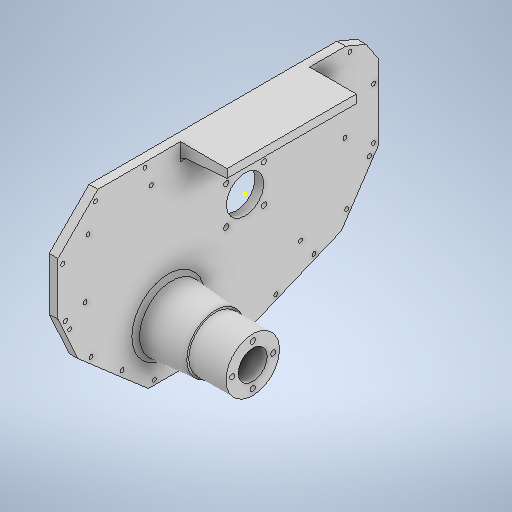
# Autodesk Inventor part: body_side_R2
Saved by Autodesk Inventor 2025.2 (Build 292293000, 293)
## iProperties
Created: 2025-04-13
Part Number: body_side_R2
Material: Generic
Document SubType Name: Modeling
Designer: Bruno
Density: 1 g/cm^3
Appearance: Default
Author: Bruno
## iProperties of the stored document body_side_R2_3DPrint.ipt
Created: 2025-05-06
Part Number: body_side_R2_3DPrint
Material: Generic
Document SubType Name: Modeling
Designer: Bruno
Density: 1 g/cm^3
Appearance: Default
Author: Bruno
Autodesk Inventor part; units mm, degrees
ref_plane "YZ Plane" through (0, 0, 0) normal (1, 0, 0) x (0, 1, 0)
ref_plane "XZ Plane" through (0, 0, 0) normal (0, 1, 0) x (-1, 0, 0)
ref_plane "XY Plane" through (0, 0, 0) normal (0, 0, 1) x (1, 0, 0)
sketch "Sketch1" plane through (0, 0, 0) normal (1, 0, 0) x (0, 1, 0)
  line L0 (0, 0) -> (-50.1885, 57.7353) construction
  line L1 (0, 0) -> (0, 3.0029) construction
  circle A0 centre (0, 0) radius 20 construction
  circle A1 centre (-14.1421, 14.1421) radius 2
  line L2 (-14.1421, 14.1421) -> (0, 0) construction
  circle A2 centre (-14.1421, -14.1421) radius 2
  circle A3 centre (14.1421, -14.1421) radius 2
  circle A4 centre (14.1421, 14.1421) radius 2
  circle A5 centre (-50.1885, 57.7353) radius 19 construction
  line L3 (-90, 0) -> (-90, 72.6202)
  line L4 (-90, 72.6202) -> (-31.0219, 140.4668)
  line L5 (-31.0219, 140.4668) -> (90, 140.4668)
  line L6 (90, 140.4668) -> (90, 0)
  line L7 (-80.2346, 83.854) -> (-64.528, 70.2004) construction
  line L8 (-90, 57.7353) -> (-69.1885, 57.7353) construction
  circle A6 centre (-34.7385, 57.7353) radius 3.55
  circle A7 centre (-50.1885, 73.1853) radius 3.55
  circle A8 centre (-65.6385, 57.7353) radius 3.55
  circle A9 centre (-50.1885, 42.2853) radius 3.55
  line L9 (-46.6385, 73.1853) -> (-46.6385, 67.9881)
  line L10 (-53.7385, 73.1853) -> (-53.7385, 67.9881)
  line L11 (-65.6385, 61.2853) -> (-60.4413, 61.2853)
  line L12 (-65.6385, 54.1853) -> (-60.4413, 54.1853)
  line L13 (-53.7385, 42.2853) -> (-53.7385, 47.4825)
  line L14 (-46.6385, 42.2853) -> (-46.6385, 47.4825)
  line L15 (-34.7385, 54.1853) -> (-39.9357, 54.1853)
  line L16 (-34.7385, 61.2853) -> (-39.9357, 61.2853)
  arc A10 (-39.9357, 61.2853) -> (-46.6385, 67.9881) centre (-50.1885, 57.7353) ccw
  arc A11 (-46.6385, 47.4825) -> (-39.9357, 54.1853) centre (-50.1885, 57.7353) ccw
  arc A12 (-53.7385, 67.9881) -> (-60.4413, 61.2853) centre (-50.1885, 57.7353) ccw
  arc A13 (-60.4413, 54.1853) -> (-53.7385, 47.4825) centre (-50.1885, 57.7353) ccw
  circle A14 centre (0, 0) radius 14
  line L17 (90, 0) -> (61.1538, -69.2308)
  line L18 (-90, 0) -> (-61.1538, -69.2308)
  circle A15 centre (0, 0) radius 46 construction
  line L19 (15, -100) -> (-15, -100)
  arc A16 (15, -100) -> (61.1538, -69.2308) centre (15, -50) ccw
  arc A17 (-61.1538, -69.2308) -> (-15, -100) centre (-15, -50) ccw
  line L20 (-50.1885, 57.7353) -> (32.543, 140.4668) construction
  line L21 (61.1538, -69.2308) -> (48.3333, -100)
  line L22 (15, -100) -> (48.3333, -100)
  line L23 (-15, -100) -> (-48.3333, -100)
  line L24 (-48.3333, -100) -> (-61.1538, -69.2308)
  point P0 (-34.7385, 61.2853)
  point P1 (-34.7385, 54.1853)
  point P2 (-46.6385, 42.2853)
  point P3 (-53.7385, 42.2853)
  point P4 (-65.6385, 54.1853)
  point P5 (-65.6385, 61.2853)
  dimension "d2" = 40
  dimension "d0" = 41
  dimension "d1" = 76.5
  dimension "d3" = 4
  dimension "d8" = 45
  dimension "d11" = 360
  dimension "d14" = 41
  dimension "d18" = 7.1
  dimension "d21" = 360
  dimension "d26" = 360
  dimension "d28" = 10.85
  dimension "d29" = 28
  dimension "d52" = 30.9
  dimension "d66" = 180
  dimension "d67" = 90
  dimension "d68" = 92
  dimension "d85" = 100
  dimension "d86" = 50
  dimension "d87" = 30
  dimension "d88" = 117
  dimension "d89" = 45
  constraints: 50 end point, 17 centre point, 17 point on circle, 10 tangent, 5 horizontal, 5 vertical, 4 coincident, 3 horizontal alignment, 3 point on line, 2 equal length, 2 line through centre, 1 equal radius, 1 perpendicular, 47 other
  measures "d0" angle of L1 L0
  measures "d1" distance of L0.end L0.start
  measures "d3" diameter of A1
  measures "d8" angle of L1 L2
  measures "d14" angle of L4 L3
  measures "d18" diameter of A6
  measures "d28" radius of A10
  measures "d29" diameter of A14
  measures "d52" distance of A9.centre A7.centre
  measures "d66" distance of L6.end L3.start
  measures "d67" distance from line of L6 A14.centre
  measures "d68" diameter of A15
  measures "d85" distance from line of L6.end L19
  measures "d86" radius of A16
  measures "d87" distance of A16.centre A17.centre
  measures "d88" distance of L20.start L20.end
  measures "d89" angle of L3 L20
extrude "Extrusion1" add sketch "Sketch1" along normal blind 6.6
sketch "Sketch2" plane through (0, 0, 0) normal (-1, 0, 0) x (0, 0, 1)
  arc A0 (54.1853, -39.9357) -> (47.4825, -46.6385) centre (57.7353, -50.1885) ccw projected
  circle A1 centre (57.7353, -50.1885) radius 21.5
  point P0 (0, 0)
  point P1 (52.1533, -40.4479)
  point P2 (48.8897, -44.3373)
  dimension "d35" = 43
  constraints: 1 centre point, 1 coincident
  measures "d35" diameter of A1
extrude "Extrusion2" add sketch "Sketch2" along normal blind 35.5
chamfer "Chamfer1" distance 3 distance2 35.5 1 edges at (0, -50.1885, 36.2353) measured on face at (0, -50.1885, 35.7353)
fillet "Fillet1" radius 3 1 edges at (0, -50.1885, 33.2354)
sketch "Sketch3" plane through (-35.5, -50.1885, 57.7353) normal (-1, 0, 0) x (0, 0, 1)
  circle A0 centre (0, 0) radius 21.5 projected
  circle A1 centre (0, 0) radius 20.05
  point P0 (-57.7353, 50.1885)
  dimension "d40" = 40.1
  constraints: 1 centre point, 1 coincident
  measures "d40" diameter of A1
extrude "Extrusion3" add sketch "Sketch3" along normal blind 28 contours A1
sketch "Sketch4" plane through (0, 0, 0) normal (1, 0, 0) x (0, 0, -1)
  arc A0 (-47.4825, -46.6385) -> (-54.1853, -39.9357) centre (-57.7353, -50.1885) ccw projected
  circle A1 centre (-57.7353, -50.1885) radius 10.85
  arc A2 (-47.4825, -46.6385) -> (-54.1853, -39.9357) centre (-57.7353, -50.1885) ccw projected
  point P0 (0, 0)
  point P1 (-54.1853, -39.9357)
  point P2 (-47.4825, -46.6385)
  point P3 (-48.8897, -44.3373)
  point P4 (-52.1533, -40.4479)
  constraints: 1 centre point, 1 coincident, 1 concentric
extrude "Extrusion4" cut sketch "Sketch4" against normal through all
sketch "Sketch5" plane through (0, 0, 0) normal (1, 0, 0) x (0, 0, -1)
  arc A0 (-42.2853, -53.7385) -> (-42.2853, -46.6385) centre (-42.2853, -50.1885) ccw projected
  circle A1 centre (-42.2853, -50.1885) radius 2
  arc A2 (-54.1853, -60.4413) -> (-47.4825, -53.7385) centre (-57.7353, -50.1885) ccw projected
  circle A3 centre (-57.7353, -34.7385) radius 2
  circle A4 centre (-73.1853, -50.1885) radius 2
  circle A5 centre (-57.7353, -65.6385) radius 2
  point P0 (0, 0)
  dimension "d45" = 4
  dimension "d48" = 360
  constraints: 4 centre point, 1 coincident, 9 other
  measures "d45" diameter of A1
extrude "Extrusion5" cut sketch "Sketch5" against normal through all
sketch "Sketch6" plane through (0, 0, 0) normal (1, 0, 0) x (0, 0, -1)
  circle A0 centre (-57.7353, -65.6385) radius 2 projected
  circle A1 centre (-57.7353, -65.6385) radius 2 projected
  arc A2 (-61.2853, -60.4413) -> (-54.1853, -60.4413) centre (-57.7353, -50.1885) ccw projected
  line L0 (-61.2853, -65.6385) -> (-61.2853, -60.4413) projected
  arc A3 (-61.2853, -65.6385) -> (-54.1853, -65.6385) centre (-57.7353, -65.6385) ccw projected
  line L1 (-54.1853, -60.4413) -> (-54.1853, -65.6385) projected
  circle A4 centre (-42.2853, -50.1885) radius 2 projected
  arc A5 (-47.4825, -53.7385) -> (-47.4825, -46.6385) centre (-57.7353, -50.1885) ccw projected
  line L2 (-42.2853, -53.7385) -> (-47.4825, -53.7385) projected
  arc A6 (-42.2853, -53.7385) -> (-42.2853, -46.6385) centre (-42.2853, -50.1885) ccw projected
  line L3 (-47.4825, -46.6385) -> (-42.2853, -46.6385) projected
  circle A7 centre (-57.7353, -34.7385) radius 2 projected
  arc A8 (-54.1853, -39.9357) -> (-61.2853, -39.9357) centre (-57.7353, -50.1885) ccw projected
  line L4 (-54.1853, -34.7385) -> (-54.1853, -39.9357) projected
  arc A9 (-54.1853, -34.7385) -> (-61.2853, -34.7385) centre (-57.7353, -34.7385) ccw projected
  line L5 (-61.2853, -39.9357) -> (-61.2853, -34.7385) projected
  circle A10 centre (-73.1853, -50.1885) radius 2 projected
  arc A11 (-67.9881, -46.6385) -> (-67.9881, -53.7385) centre (-57.7353, -50.1885) ccw projected
  line L6 (-73.1853, -46.6385) -> (-67.9881, -46.6385) projected
  arc A12 (-73.1853, -46.6385) -> (-73.1853, -53.7385) centre (-73.1853, -50.1885) ccw projected
  line L7 (-67.9881, -53.7385) -> (-73.1853, -53.7385) projected
  line L8 (-42.2853, -53.7385) -> (-47.4825, -53.7385) projected
  arc A13 (-42.2853, -53.7385) -> (-42.2853, -46.6385) centre (-42.2853, -50.1885) ccw projected
  line L9 (-47.4825, -46.6385) -> (-42.2853, -46.6385) projected
  arc A14 (-47.4825, -53.7385) -> (-47.4825, -46.6385) centre (-57.7353, -50.1885) ccw projected
  arc A15 (-61.2853, -60.4413) -> (-54.1853, -60.4413) centre (-57.7353, -50.1885) ccw projected
  line L10 (-61.2853, -65.6385) -> (-61.2853, -60.4413) projected
  arc A16 (-61.2853, -65.6385) -> (-54.1853, -65.6385) centre (-57.7353, -65.6385) ccw projected
  line L11 (-54.1853, -60.4413) -> (-54.1853, -65.6385) projected
  arc A17 (-67.9881, -46.6385) -> (-67.9881, -53.7385) centre (-57.7353, -50.1885) ccw projected
  line L12 (-73.1853, -46.6385) -> (-67.9881, -46.6385) projected
  arc A18 (-73.1853, -46.6385) -> (-73.1853, -53.7385) centre (-73.1853, -50.1885) ccw projected
  line L13 (-67.9881, -53.7385) -> (-73.1853, -53.7385) projected
  arc A19 (-54.1853, -39.9357) -> (-61.2853, -39.9357) centre (-57.7353, -50.1885) ccw projected
  line L14 (-54.1853, -34.7385) -> (-54.1853, -39.9357) projected
  arc A20 (-54.1853, -34.7385) -> (-61.2853, -34.7385) centre (-57.7353, -34.7385) ccw projected
  line L15 (-61.2853, -39.9357) -> (-61.2853, -34.7385) projected
  arc A21 (-61.2853, -60.4413) -> (-54.1853, -60.4413) centre (-57.7353, -50.1885) ccw projected
  line L16 (-61.2853, -65.6385) -> (-61.2853, -60.4413) projected
  arc A22 (-61.2853, -65.6385) -> (-54.1853, -65.6385) centre (-57.7353, -65.6385) ccw projected
  line L17 (-54.1853, -60.4413) -> (-54.1853, -65.6385) projected
  arc A23 (-67.9881, -46.6385) -> (-67.9881, -53.7385) centre (-57.7353, -50.1885) ccw projected
  line L18 (-73.1853, -46.6385) -> (-67.9881, -46.6385) projected
  arc A24 (-73.1853, -46.6385) -> (-73.1853, -53.7385) centre (-73.1853, -50.1885) ccw projected
  line L19 (-67.9881, -53.7385) -> (-73.1853, -53.7385) projected
  point P0 (0, 0)
extrude "Extrusion6" cut sketch "Sketch6" against normal blind 20.5 contours A0 | A2 L1 A3 L0 | A4 | A5 L3 A6 L2 | A8 L5 A9 L4 | A11 L7 A12 L6
sketch "Sketch7" plane through (6.6, 0, 0) normal (1, 0, 0) x (0, 0, -1)
  circle A0 centre (0, 0) radius 14 projected
  line L0 (0, 14) -> (0, 32) construction
  line L1 (0, 32) -> (3, 32) construction
  line L2 (0, 38) -> (3, 38) construction
  arc A1 (3, 32) -> (3, 38) centre (3, 35) ccw construction
  line L3 (0, 32) -> (-3, 32) construction
  line L4 (0, 38) -> (-3, 38) construction
  arc A2 (-3, 38) -> (-3, 32) centre (-3, 35) ccw construction
  line L5 (-3, 39.5) -> (0, 39.5)
  line L6 (0, 39.5) -> (3, 39.5)
  arc A3 (3, 30.5) -> (3, 39.5) centre (3, 35) ccw
  line L7 (3, 30.5) -> (0, 30.5)
  line L8 (0, 30.5) -> (-3, 30.5)
  arc A4 (-3, 39.5) -> (-3, 30.5) centre (-3, 35) ccw
  dimension "d55" = 18
  dimension "d56" = 3
  dimension "d57" = 6
  dimension "d58" = 1.5
  constraints: 18 end point, 8 point on circle, 4 centre point, 3 symmetric about line, 2 horizontal, 2 tangent, 2 vertical alignment, 1 vertical, 7 other
  measures "d55" distance of L0.start L0.end
  measures "d56" distance of L0.end L1.end
  measures "d57" distance between parallel lines of L2 L1
  measures "d58" distance between parallel lines of L4 L5
extrude "Extrusion7" cut sketch "Sketch7" against normal through all contours L5 L6 A3 L7 L8 A4
sketch "Sketch8" plane through (6.6, 0, 0) normal (1, 0, 0) x (0, 0, -1)
  circle A0 centre (-30, 22) radius 2.225
  circle A1 centre (0, 0) radius 14 projected
  line L0 (0, 0) -> (-5.1199, 0) construction
  line L1 (0, 0) -> (0, 4.2837) construction
  circle A2 centre (-30, -22) radius 2.225
  circle A3 centre (30, 22) radius 2.225
  circle A4 centre (30, -22) radius 2.225
  dimension "d61" = 4.45
  dimension "d62" = 30
  dimension "d63" = 22
  constraints: 4 centre point, 4 end point, 3 symmetric about line, 1 horizontal, 1 vertical, 3 other
  measures "d61" diameter of A0
  measures "d62" horizontal distance of A0.centre L0.start
  measures "d63" vertical distance of A0.centre L0.start
extrude "Extrusion8" cut sketch "Sketch8" against normal blind 6 contours A0 | A2 | A3 | A4
sketch "Sketch13" plane through (6.6, 0, 0) normal (1, 0, 0) x (0, 0, -1)
  circle A0 centre (0, 0) radius 14 projected
  circle A1 centre (0, 0) radius 46 construction
  line L0 (0, 103.5) -> (0, 58.5) construction
  line L1 (-26, 58.5) -> (26, 58.5)
  line L2 (25.1057, 48.5) -> (-25.1057, 48.5) construction
  line L3 (0, 46) -> (0, 48.5) construction
  line L4 (0, 90) -> (-140.4668, 90) projected
  line L5 (-26, 58.5) -> (-26, 90)
  line L6 (26, 58.5) -> (26, 79.1667)
  line L7 (-140.4668, 90) -> (-140.4668, -31.0219) projected
  line L8 (26, 58.5) -> (75.6, 58.5)
  line L9 (-26, 58.5) -> (-140.4668, 58.5)
  line L10 (100, 48.3333) -> (0, 90) projected
  dimension "d90" = 92
  dimension "d91" = 45
  dimension "d92" = 52
  dimension "d93" = 10
  dimension "d94" = 2.5
  constraints: 16 end point, 4 vertical alignment, 3 horizontal, 3 point on line, 3 vertical, 2 midpoint, 2 perpendicular, 1 coincident, 2 other
  measures "d91" distance of L0.start L0.end
  measures "d92" distance of L1.start L1.end
  measures "d93" distance between parallel lines of L1 L2
  measures "d94" distance of L3.start L3.end
extrude "Extrusion9" cut sketch "Sketch13" against normal blind 10 contours L5 L4 L10 L6 L1 | L9 L7 L4 L5 | L6 L10 L8
sketch "Sketch15" plane through (0, 0, 0) normal (-1, 0, 0) x (0, 0, 1)
  point P0 (0, 0)
chamfer "Chamfer2" distance 30 angle 45 2 edges at (3.3, -48.3333, -100) (3.3, 58.5, 140.4668)
chamfer "Chamfer3" distance 20 angle 45 1 edges at (3.3, -31.0219, 140.4668)
chamfer "Chamfer4" distance 10 angle 45 1 edges at (3.3, 48.3333, -100)
sketch "Sketch16" plane through (0, 0, 0) normal (-1, 0, 0) x (0, 0, 1)
  line L0 (-100, 38.3333) -> (-90.7692, 52.1795) projected
  line L1 (-100, -18.3333) -> (-100, 38.3333) projected
  line L2 (-72.3077, -59.8718) -> (-100, -18.3333) projected
  line L3 (0, -90) -> (-72.3077, -59.8718) projected
  line L4 (72.6202, -90) -> (0, -90) projected
  line L5 (125.3726, -44.143) -> (72.6202, -90) projected
  line L6 (140.4668, -11.0219) -> (125.3726, -44.143) projected
  line L7 (140.4668, 28.5) -> (140.4668, -11.0219) projected
  line L8 (110.4668, 58.5) -> (140.4668, 28.5) projected
  line L9 (110.4668, 58.5) -> (-75.6, 58.5) projected
  line L10 (-90.7692, 52.1795) -> (-75.6, 58.5) projected
  arc A0 (3, 30.5) -> (3, 39.5) centre (3, 35) ccw projected
  line L11 (3, 30.5) -> (-3, 30.5) projected
  arc A1 (-3, 39.5) -> (-3, 30.5) centre (-3, 35) ccw projected
  line L12 (-3, 39.5) -> (3, 39.5) projected
  circle A2 centre (14.1421, -14.1421) radius 2 projected
  circle A3 centre (-14.1421, -14.1421) radius 2 projected
  circle A4 centre (-14.1421, 14.1421) radius 2 projected
  circle A5 centre (14.1421, 14.1421) radius 2 projected
  circle A6 centre (0, 0) radius 14 projected
  circle A7 centre (57.7353, -50.1885) radius 27.2572 projected
  line L13 (-90.7692, 52.1795) -> (116.7873, 52.1795)
  circle A8 centre (0, 0) radius 46 construction
  circle A9 centre (0, 0) radius 48.5
  line L14 (-48.5, 0) -> (-48.5, 58.5)
  line L15 (48.5, 0) -> (48.5, 58.5)
  point P0 (48.5, 52.1795)
  point P1 (-48.5, 52.1795)
  dimension "d115" = 92
  dimension "d116" = 2.5
  constraints: 6 end point, 3 point on line, 2 centre point, 2 coincident, 2 perpendicular, 2 point on circle, 2 tangent, 1 horizontal
  measures "d115" diameter of A8
  measures "d116" radial gap between concentric circles of A8 A9
extrude "Extrusion11" add sketch "Sketch16" along normal blind 35 contours L14 L9 L15 L13
sketch "Sketch18" plane through (6.6, 0, 0) normal (1, 0, 0) x (0, 0, -1)
  circle A0 centre (96.475, 23.7415) radius 1.5 projected
  circle A1 centre (96.475, 23.7415) radius 1.5 projected
  circle A2 centre (96.475, -14.8083) radius 1.5 projected
  circle A3 centre (93.4135, -21.8583) radius 1.5 projected
  circle A4 centre (76.1956, -47.6852) radius 1.5 projected
  circle A5 centre (51.6799, -64.648) radius 1.5 projected
  circle A6 centre (23.0276, -76.5864) radius 1.5 projected
  circle A7 centre (-6.0346, -86.475) radius 1.5 projected
  circle A8 centre (-37.0746, -86.475) radius 1.5 projected
  circle A9 centre (-68.1146, -86.475) radius 1.5 projected
  circle A10 centre (-92.3227, -68.2022) radius 1.5 projected
  circle A11 centre (-115.7488, -47.8382) radius 1.5 projected
  circle A12 centre (-131.6545, -21.8583) radius 1.5 projected
  circle A13 centre (-134.8674, -14.8083) radius 1.5 projected
  circle A14 centre (-136.9418, 23.2911) radius 1.5 projected
  circle A15 centre (-112.3337, 51.6479) radius 1.5 projected
  circle A16 centre (-75.162, 54.975) radius 1.5 projected
  circle A17 centre (-36.6122, 54.975) radius 1.5 projected
  circle A18 centre (1.9376, 54.975) radius 1.5 projected
  circle A19 centre (40.4874, 54.975) radius 1.5 projected
  circle A20 centre (78.7186, 53.3818) radius 1.5 projected
  circle A21 centre (-134.8674, -14.8083) radius 1.65
  point P0 (0, 0)
  dimension "d117" = 3.3
  constraints: 1 centre point, 1 coincident
  measures "d117" diameter of A21
extrude "Extrusion12" cut sketch "Sketch18" against normal through all contours A0 | A2 | A3 | A4 | A5 | A6 | A7 | A8 | A9 | A10 | A11 | A12 | A13 | A14 | A15 | A16 | A20 | A21
chamfer "Chamfer5" distance 3 distance2 35 1 edges at (0, 52.1795, 0) measured on face at (0, 51.6795, 0)
fillet "Fillet5" radius 4 1 edges at (0, 49.1796, 0)
sketch "Sketch19" plane through (6.6, 0, 0) normal (1, 0, 0) x (0, 0, -1)
  circle A0 centre (60.0011, 43.3256) radius 2.225 projected
  circle A1 centre (41.5764, -50.8737) radius 2.225 projected
  circle A2 centre (74.9972, -0.7443) radius 2.225 projected
  circle A3 centre (96.475, 23.7415) radius 2.8 projected
  circle A4 centre (51.6799, -64.648) radius 2.8 projected
  circle A5 centre (96.475, -14.8083) radius 2.8 projected
  circle A6 centre (78.7186, 53.3818) radius 2.8 projected
  circle A7 centre (76.1956, -47.6852) radius 2.8 projected
  circle A8 centre (93.4135, -21.8583) radius 2.8 projected
  arc A9 (30.8564, -39.3432) -> (27.0276, -47.2118) centre (37.0276, -47.2118) ccw projected
  line L0 (27.0276, -78.7385) -> (27.0276, -47.2118) projected
  line L1 (72.3077, -59.8718) -> (27.0276, -78.7385) projected
  line L2 (100, -18.3333) -> (72.3077, -59.8718) projected
  line L3 (100, 38.3333) -> (100, -18.3333) projected
  line L4 (90.7692, 52.1795) -> (100, 38.3333) projected
  line L5 (75.6, 58.5) -> (90.7692, 52.1795) projected
  line L6 (48.5, 58.5) -> (75.6, 58.5) projected
  line L7 (48.5, 45.5077) -> (48.5, 58.5) projected
  line L8 (32.8444, 41.8922) -> (48.5, 45.5077) projected
  arc A10 (32.8444, 41.8922) -> (32.0139, 38.4072) centre (33.2944, 39.9435) ccw projected
  arc A11 (30.8564, -39.3432) -> (32.0139, 38.4072) centre (0, 0) ccw projected
  circle A12 centre (-120.1367, -10.0647) radius 2.225 projected
  circle A13 centre (-117.9117, 32.9479) radius 2.225 projected
  circle A14 centre (-70.353, 41.1006) radius 2.225 projected
  circle A15 centre (-136.9418, 23.2911) radius 2.8 projected
  circle A16 centre (-112.3337, 51.6479) radius 2.8 projected
  circle A17 centre (-134.8674, -14.8083) radius 2.8 projected
  circle A18 centre (-75.162, 54.975) radius 2.8 projected
  circle A19 centre (-131.6545, -21.8583) radius 2.8 projected
  arc A20 (-42.1883, 31.8997) -> (-35.8142, 34.8905) centre (-42.977, 41.8686) ccw projected
  arc A21 (-32.0139, 38.4072) -> (-35.8142, 34.8905) centre (0, 0) ccw projected
  arc A22 (-32.0139, 38.4072) -> (-32.8444, 41.8922) centre (-33.2944, 39.9435) ccw projected
  line L9 (-48.5, 45.5077) -> (-32.8444, 41.8922) projected
  line L10 (-48.5, 58.5) -> (-48.5, 45.5077) projected
  line L11 (-110.4668, 58.5) -> (-48.5, 58.5) projected
  line L12 (-140.4668, 28.5) -> (-110.4668, 58.5) projected
  line L13 (-140.4668, -11.0219) -> (-140.4668, 28.5) projected
  line L14 (-125.3726, -44.143) -> (-140.4668, -11.0219) projected
  line L15 (-87.7648, 23.7979) -> (-125.3726, -44.143) projected
  arc A23 (-79.8044, 28.9239) -> (-87.7648, 23.7979) centre (-79.0157, 18.955) ccw projected
  line L16 (-42.1883, 31.8997) -> (-79.8044, 28.9239) projected
  circle A24 centre (-70.353, 41.1006) radius 1.5
  circle A25 centre (-117.9117, 32.9479) radius 1.5
  circle A26 centre (-120.1367, -10.0647) radius 1.5
  circle A27 centre (60.0011, 43.3256) radius 1.5
  circle A28 centre (74.9972, -0.7443) radius 1.5
  circle A29 centre (41.5764, -50.8737) radius 1.5
  point P0 (0, 0)
  dimension "d124" = 3
  dimension "d125" = 3
  dimension "d126" = 3
  dimension "d127" = 3
  dimension "d128" = 3
  dimension "d129" = 3
  constraints: 6 centre point, 6 coincident
  measures "d124" diameter of A24
  measures "d125" diameter of A25
  measures "d126" diameter of A26
  measures "d127" diameter of A27
  measures "d128" diameter of A28
  measures "d129" diameter of A29
extrude "Extrusion13" cut sketch "Sketch19" against normal through all contours A24 | A25 | A26 | A27 | A28 | A29
sketch "Sketch20" plane through (6.6, 0, 0) normal (1, 0, 0) x (0, 0, -1)
  circle A0 centre (-117.9117, 32.9479) radius 1.5 projected
  circle A1 centre (-117.9117, 32.9479) radius 2.8
  circle A2 centre (-70.353, 41.1006) radius 1.5 projected
  circle A3 centre (-70.353, 41.1006) radius 2.8
  circle A4 centre (-120.1367, -10.0647) radius 1.5 projected
  circle A5 centre (-120.1367, -10.0647) radius 2.8
  circle A6 centre (60.0011, 43.3256) radius 1.5 projected
  circle A7 centre (60.0011, 43.3256) radius 2.8
  circle A8 centre (74.9972, -0.7443) radius 1.5 projected
  circle A9 centre (74.9972, -0.7443) radius 2.8
  circle A10 centre (41.5764, -50.8737) radius 1.5 projected
  circle A11 centre (41.5764, -50.8737) radius 2.8
  point P0 (0, 0)
  dimension "d132" = 5.6
  dimension "d133" = 5.6
  dimension "d134" = 5.6
  dimension "d135" = 5.6
  dimension "d136" = 5.6
  dimension "d137" = 5.6
  constraints: 6 centre point, 6 coincident
  measures "d132" diameter of A1
  measures "d133" diameter of A3
  measures "d134" diameter of A5
  measures "d135" diameter of A7
  measures "d136" diameter of A9
  measures "d137" diameter of A11
extrude "Extrusion14" cut sketch "Sketch20" against normal blind 3 contours A1 | A3 | A4 | A5 | A6 | A7 | A8 | A9 | A11
mirror "Mirror1" about plane through (0, 0, 0) normal (1, 0, 0) remove original yes
sketch "Sketch21" plane through (-6.6, -18.3333, -100) normal (-1, 0, 0) x (0, 0, 1)
  circle A0 centre (85.8579, 32.4755) radius 2 projected
  circle A1 centre (85.8579, 32.4755) radius 3.55
  circle A2 centre (114.1421, 32.4755) radius 2 projected
  circle A3 centre (114.1421, 32.4755) radius 3.55
  circle A4 centre (114.1421, 4.1912) radius 2 projected
  circle A5 centre (114.1421, 4.1912) radius 3.55
  circle A6 centre (85.8579, 4.1912) radius 2 projected
  circle A7 centre (85.8579, 4.1912) radius 3.55
  point P0 (100, 18.3333)
  dimension "d140" = 7.1
  dimension "d141" = 7.1
  dimension "d142" = 7.1
  dimension "d143" = 7.1
  constraints: 4 centre point, 4 coincident
  measures "d140" diameter of A1
  measures "d141" diameter of A3
  measures "d142" diameter of A5
  measures "d143" diameter of A7
extrude "Extrusion15" cut sketch "Sketch21" against normal blind 2 contours A0 | A1 | A2 | A3 | A4 | A5 | A6 | A7
sketch "Sketch22" plane through (20.5, -39.9357, 61.2853) normal (-1, 0, 0) x (0, 0, 1)
  circle A0 centre (-3.55, 5.1972) radius 2 projected
  line L0 (0, 0) -> (0, 5.1972) projected
  arc A1 (0, 5.1972) -> (-7.1, 5.1972) centre (-3.55, 5.1972) ccw projected
  line L1 (-7.1, 5.1972) -> (-7.1, 0) projected
  arc A2 (0, 0) -> (-7.1, 0) centre (-3.55, -10.2528) ccw projected
  circle A3 centre (-19, -10.2528) radius 2 projected
  line L2 (-13.8028, -6.7028) -> (-19, -6.7028) projected
  arc A4 (-19, -6.7028) -> (-19, -13.8028) centre (-19, -10.2528) ccw projected
  line L3 (-19, -13.8028) -> (-13.8028, -13.8028) projected
  arc A5 (-13.8028, -6.7028) -> (-13.8028, -13.8028) centre (-3.55, -10.2528) ccw projected
  circle A6 centre (-3.55, -25.7028) radius 2 projected
  line L4 (-7.1, -20.5056) -> (-7.1, -25.7028) projected
  arc A7 (-7.1, -25.7028) -> (0, -25.7028) centre (-3.55, -25.7028) ccw projected
  line L5 (0, -25.7028) -> (0, -20.5056) projected
  arc A8 (-7.1, -20.5056) -> (0, -20.5056) centre (-3.55, -10.2528) ccw projected
  line L6 (6.7028, -13.8028) -> (11.9, -13.8028) projected
  arc A9 (11.9, -13.8028) -> (11.9, -6.7028) centre (11.9, -10.2528) ccw projected
  line L7 (11.9, -6.7028) -> (6.7028, -6.7028) projected
  arc A10 (6.7028, -13.8028) -> (6.7028, -6.7028) centre (-3.55, -10.2528) ccw projected
  circle A11 centre (11.9, -10.2528) radius 2 projected
  line L8 (-7.1, 0.5972) -> (0, 0.5972)
  line L9 (-7.1, 3.1972) -> (0, 3.1972)
  line L10 (-6.483, 7.1972) -> (-0.617, 7.1972)
  circle A12 centre (-3.55, 5.1972) radius 2 projected
  arc A13 (0, 0) -> (-7.1, 0) centre (-3.55, -10.2528) ccw projected
  line L11 (-21, -13.1858) -> (-21, -7.3198)
  line L12 (-17, -13.8028) -> (-17, -6.7028)
  line L13 (-14.4, -13.8028) -> (-14.4, -6.7028)
  line L14 (-0.617, -27.7028) -> (-6.483, -27.7028)
  line L15 (0, -23.7028) -> (-7.1, -23.7028)
  line L16 (0, -21.1028) -> (-7.1, -21.1028)
  line L17 (13.9, -7.3198) -> (13.9, -13.1858)
  line L18 (9.9, -6.7028) -> (9.9, -13.8028)
  line L19 (7.3, -6.7028) -> (7.3, -13.8028)
  point P0 (-61.2853, 39.9357)
  point P1 (-6.483, -27.7028)
  point P2 (-0.617, -27.7028)
  point P3 (-7.1, -21.1028)
  point P4 (-7.1, -23.7028)
  point P5 (0, -23.7028)
  point P6 (0, -21.1028)
  point P7 (13.9, -13.1858)
  point P8 (13.9, -7.3198)
  point P9 (7.3, -13.8028)
  point P10 (9.9, -13.8028)
  point P11 (9.9, -6.7028)
  point P12 (7.3, -6.7028)
  point P13 (-14.4, -6.7028)
  point P14 (-17, -6.7028)
  point P15 (-17, -13.8028)
  point P16 (-14.4, -13.8028)
  point P17 (-21, -7.3198)
  dimension "d148" = 360
  constraints: 24 end point, 4 point on line, 3 tangent, 2 parallel, 2 point on circle, 1 perpendicular, 37 other
extrude "Extrusion16" add sketch "Sketch22" along normal blind 0.2 contours L10 A1 | L9 L0 L8 L1 | L12 L2 L13 L3 | L11 A4 | L15 L4 L16 L5 | L14 A7 | L19 L7 L18 L6 | L17 A9
sketch "Sketch23" plane through (-4.6, 14.1421, -14.1421) normal (-1, 0, 0) x (0, 0, 1)
  circle A0 centre (0, 0) radius 2 projected
  circle A1 centre (0, 0) radius 3.55 projected
  circle A2 centre (0, -28.2843) radius 2 projected
  circle A3 centre (0, -28.2843) radius 3.55 projected
  circle A4 centre (28.2843, -28.2843) radius 2 projected
  circle A5 centre (28.2843, -28.2843) radius 3.55 projected
  circle A6 centre (28.2843, 0) radius 2 projected
  circle A7 centre (28.2843, 0) radius 3.55 projected
  line L0 (-2, 2.933) -> (-2, -31.2173)
  line L1 (2, 2.933) -> (2, -31.2173)
  line L2 (26.2843, 2.933) -> (26.2843, -31.2173)
  line L3 (30.2843, -31.2173) -> (30.2843, 2.933)
  point P0 (14.1421, -14.1421)
  point P1 (30.2843, -2.933)
  point P2 (26.2843, -2.933)
  point P3 (30.2843, -25.3513)
  point P4 (26.2843, -25.3513)
  point P5 (2, -25.3513)
  point P6 (-2, -25.3513)
  point P7 (2, -2.933)
  point P8 (-2, -2.933)
  constraints: 8 end point, 8 point on circle, 4 tangent, 3 parallel, 1 vertical
extrude "Extrusion17" add sketch "Sketch23" along normal blind 0.2 contours L1 A1 | L0 A1 | A3 L1 | L0 A3 | L3 A5 | L2 A5 | L3 A7 | A7 L2
sketch "Sketch24" plane through (-3.6, 43.3256, -60.0011) normal (-1, 0, 0) x (0, 0, 1)
  circle A0 centre (0, 0) radius 1.5 projected
  circle A1 centre (0, 0) radius 2.8 projected
  circle A2 centre (-14.9961, -44.0699) radius 1.5 projected
  circle A3 centre (-14.9961, -44.0699) radius 2.8 projected
  circle A4 centre (18.4247, -94.1993) radius 2.8 projected
  circle A5 centre (18.4247, -94.1993) radius 1.5 projected
  circle A6 centre (180.1379, -53.3903) radius 1.5 projected
  circle A7 centre (180.1379, -53.3903) radius 2.8 projected
  circle A8 centre (177.9129, -10.3777) radius 2.8 projected
  circle A9 centre (177.9129, -10.3777) radius 1.5 projected
  circle A10 centre (130.3541, -2.225) radius 2.8 projected
  circle A11 centre (130.3541, -2.225) radius 1.5 projected
  line L0 (128.8541, 0.1393) -> (128.8541, -4.5893)
  line L1 (131.8541, 0.1393) -> (131.8541, -4.5893)
  line L2 (176.4129, -8.0134) -> (176.4129, -12.742)
  line L3 (179.4129, -8.0134) -> (179.4129, -12.742)
  line L4 (178.6379, -51.026) -> (178.6379, -55.7547)
  line L5 (181.6379, -51.026) -> (181.6379, -55.7547)
  circle A12 centre (180.1379, -53.3903) radius 1.5 projected
  circle A13 centre (177.9129, -10.3777) radius 1.5 projected
  line L6 (-1.5, 2.3643) -> (-1.5, -2.3643)
  line L7 (1.5, 2.3643) -> (1.5, -2.3643)
  line L8 (-16.4961, -41.7056) -> (-16.4961, -46.4342)
  line L9 (-13.4961, -41.7056) -> (-13.4961, -46.4342)
  line L10 (16.9247, -91.835) -> (16.9247, -96.5637)
  line L11 (19.9247, -91.835) -> (19.9247, -96.5637)
  circle A14 centre (-14.9961, -44.0699) radius 1.5 projected
  circle A15 centre (0, 0) radius 1.5 projected
  point P0 (60.0011, -43.3256)
  constraints: 24 end point, 24 point on circle, 12 tangent, 8 parallel, 4 vertical
extrude "Extrusion18" add sketch "Sketch24" along normal blind 0.2 contours L7 A1 | L6 A1 | L9 A3 | L8 A3 | A4 L11 | L10 A4 | L5 A7 | L4 A7 | A8 L3 | L2 A8 | A10 L1 | L0 A10
body "Solid1"
